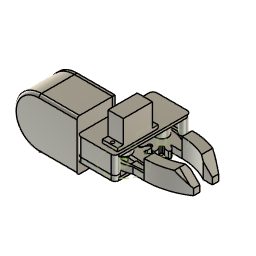
TRARM02_Link4_Gripper (Autodesk Fusion 360 design; units mm, degrees)
description: Spur Gear; Module: 2.5; Num Teeth: 12; Pressure Angle: 20.0; Backlash: 0.00 mm
Autodesk Fusion 360 part; units mm, degrees
(part 1 of 2)
sketch "스케치1" plane through (0, 0, 0) normal (0, 0, 1) x (1, 0, 0) in component "TRARM02_Link4A_30x40x2 v1"
  line L0 (20, 30) -> (20, 0)
  line L1 (-20, 30) -> (-20, 0)
  arc A0 (-20, 0) -> (20, 0) centre (0, 0) ccw
  line L2 (-20, 30) -> (20, 30)
  dimension "d1" = 40
  dimension "d128" = 30
  dimension "d129" = 20
  constraint coincident A0.centre origin
  constraint tangent L0 A0
  constraint vertical L0
  constraint parallel L0 L1
  constraint horizontal L0.start L1.start
  measures "d1" diameter of A0
  measures "d128" vertical distance of A0.centre L1.start
  measures "d129" distance of A0.centre L1
extrude "돌출1" add sketch "스케치1" along normal blind 2 makes body 1 in component "TRARM02_Link4A_30x40x2 v1"
sketch "스케치2" plane through (0, 0, 2) normal (0, 0, 1) x (-1, 0, 0) in component "TRARM02_Link4A_30x40x2 v1"
  circle A0 centre (0, 8.75) radius 1.1
  circle A1 centre (0, -19.05) radius 1.1
  line L0 (6.1, -16.65) -> (-6.1, -16.65)
  line L1 (-6.1, -16.65) -> (-6.1, 6.35)
  line L2 (-6.1, 6.35) -> (6.1, 6.35)
  line L3 (6.1, 6.35) -> (6.1, -16.65)
  dimension "d7" = 2.2
  dimension "d8" = 27.8
  dimension "d9" = 8.75
  dimension "d11" = 23
  dimension "d12" = 2.4
  dimension "d13" = 12.2
  dimension "d14" = 6.1
  constraint equal A0 A1
  constraint horizontal L0
  constraint vertical L1
  constraint horizontal L2
  constraint vertical L3
  constraint vertical origin A0.centre
  constraint vertical origin A1.centre
  measures "d7" diameter of A0
  measures "d8" distance of A0.centre A1.centre
  measures "d9" distance of origin A0.centre
  measures "d11" distance of L0.end L1.end
  measures "d12" vertical distance of A1.centre L0.end
  measures "d13" distance of L0.start L0.end
  measures "d14" horizontal distance of origin L1.end
extrude "돌출2" cut sketch "스케치2" against normal blind 2 bodies 1 in component "TRARM02_Link4A_30x40x2 v1"
chamfer "챔퍼2" distance 1.5 angle 45 2 edges at (1.0256, 19.4478, 0) (1.0256, -8.3522, 0) on bodies 1 in component "TRARM02_Link4A_30x40x2 v1"
sketch "스케치14" plane through (0, 0, 2) normal (0, 0, 1) x (-1, 0, 0) in component "TRARM02_Link4A_30x40x2 v1"
  line L0 (20, -30) -> (20, 0) construction
  line L1 (-20, 0) -> (-20, -30) construction
  arc A0 (20, 0) -> (-20, 0) centre (0, 0) ccw construction
  line L2 (19, -29) -> (19, 0)
  arc A1 (19, 0) -> (-19, 0) centre (0, 0) ccw
  line L3 (-19, 0) -> (-19, -29)
  line L4 (-15, -6) -> (-18, -6)
  line L5 (15, -6) -> (18, -6)
  line L6 (15, 0) -> (18, 0)
  arc A2 (15, 0) -> (15, -6) centre (15, -3) ccw
  line L7 (18, -28) -> (18, -6)
  line L8 (-18, -6) -> (-18, -28)
  line L9 (-15, 0) -> (-18, 0)
  arc A3 (18, 0) -> (-18, 0) centre (0, 0) ccw
  arc A4 (-15, -6) -> (-15, 0) centre (-15, -3) ccw
  line L10 (-20, -30) -> (20, -30)
  line L11 (18, -28) -> (-18, -28)
  line L12 (19, -29) -> (-19, -29)
  dimension "d112" = 3
  dimension "d113" = 3
  dimension "d120" = 3
  dimension "d121" = 1
  dimension "d124" = 6
  dimension "d125" = 6
  dimension "d126" = 3
  dimension "d130" = 1
  dimension "d131" = 1
  constraint coincident L6.end L7
  constraint perpendicular L6 L7
  constraint coincident L6 A2.start
  constraint horizontal L5
  constraint vertical L6.start A2.centre
  constraint coincident L6.start A2.start
  constraint horizontal L4
  constraint horizontal L9
  constraint vertical L8
  constraint equal L4 L9
  constraint vertical L4.end L9.end
  constraint coincident A0.centre L6
  constraint coincident A0.centre L9
  constraint concentric A0 A3
  constraint concentric A0 A1
  constraint tangent L2 A1
  constraint tangent A1 L3
  constraint vertical L7
  constraint horizontal L12
  constraint horizontal L11
  measures "d112" distance of L5.start L5.end
  measures "d113" distance of L4.start L4.end
  measures "d120" distance of L6.start L6.end
  measures "d121" distance of L3 L8
  measures "d124" distance of A0.centre L5
  measures "d125" distance of A0.centre L4
  measures "d126" radius of A4
  measures "d130" distance of L11 L12
  measures "d131" distance of L10 L12
extrude "돌출15" add sketch "스케치14" along normal blind 2 bodies 1 in component "TRARM02_Link4A_30x40x2 v1"
sketch "스케치16" plane through (0, 0, 4) normal (0, 0, 1) x (-1, 0, 0) in component "TRARM02_Link4A_30x40x2 v1"
  circle A0 centre (-15, -3) radius 1.5
  circle A1 centre (15, -3) radius 1.5
  arc A2 (15, 0) -> (15, -6) centre (15, -3) ccw
  arc A3 (-15, -6) -> (-15, 0) centre (-15, -3) ccw
  dimension "d106" = 3
  constraint equal A0 A1
  constraint concentric A1 A2
  constraint concentric A0 A3
  measures "d106" diameter of A0
extrude "돌출17" cut sketch "스케치16" against normal blind 4 bodies 1 in component "TRARM02_Link4A_30x40x2 v1"
chamfer "챔퍼4" distance 2 angle 45 1 edges at (16.3985, 3.5424, 0) on bodies 1 in component "TRARM02_Link4A_30x40x2 v1"
chamfer "챔퍼4" distance 2 angle 45 1 edges at (-13.6015, 3.5424, 0) on bodies 1 in component "TRARM02_Link4A_30x40x2 v1"
move_body "이동1" bodies 1 to x (0, -1, 0) y (1, 0, 0) z (0, 0, 1) at (0, 0, 0) in component "TRARM02_Link4A_30x40x2 v1"
sketch "스케치1 (2)" plane through (0, 0, 0) normal (0, 0, 1) x (1, 0, 0) in component "TRARM02_Link4B_30x40x28 v1"
  line L0 (20, 30) -> (20, 0)
  line L1 (-20, 30) -> (-20, 0)
  arc A0 (-20, 0) -> (20, 0) centre (0, 0) ccw
  line L2 (-20, 30) -> (20, 30)
  dimension "d1_1" = 40
  dimension "d144" = 30
  constraint coincident A0.centre origin
  constraint tangent L0 A0
  constraint vertical L0
  constraint parallel L0 L1
  constraint horizontal L0.start L1.start
  measures "d1_1" diameter of A0
  measures "d144" vertical distance of A0.centre L1.start
extrude "돌출1'" add sketch "스케치1 (2)" along normal blind 2 separate body makes body 2 in component "TRARM02_Link4B_30x40x28 v1"
sketch "스케치14 (2)" plane through (0, 0, 2) normal (0, 0, 1) x (-1, 0, 0) in component "TRARM02_Link4B_30x40x28 v1"
  line L0 (20, -30) -> (20, 0)
  line L1 (-20, 0) -> (-20, -30)
  arc A0 (20, 0) -> (-20, 0) centre (0, 0) ccw
  arc A1 (19, 0) -> (-19, 0) centre (0, 0) ccw
  line L2 (15, -6) -> (19, -6)
  line L3 (15, 0) -> (19, 0)
  arc A2 (15, 0) -> (15, -6) centre (15, -3) ccw
  line L4 (-15, -6) -> (-19, -6)
  arc A3 (-15, -6) -> (-15, 0) centre (-15, -3) ccw
  line L5 (19, -29) -> (19, -6)
  line L6 (-19, -6) -> (-19, -29)
  line L7 (-15, 0) -> (-19, 0)
  line L8 (-20, -30) -> (20, -30)
  line L9 (20, -30) -> (-20, -30)
  line L10 (19, -29) -> (-19, -29)
  dimension "d111_1" = 15
  dimension "d112_1" = 6
  dimension "d114" = 3
  dimension "d132" = 4
  dimension "d133" = 4
  dimension "d134" = 4
  dimension "d135" = 1
  dimension "d136" = 4
  dimension "d142" = 1
  dimension "d143" = 19
  dimension "d145" = 1
  constraint concentric A0 A1
  constraint equal A2 A3
  constraint horizontal A2.centre A3.centre
  constraint horizontal L7
  constraint vertical L6
  constraint horizontal L4
  constraint vertical L5
  constraint horizontal L3
  constraint coincident A1.start L3.end
  constraint horizontal L2
  constraint coincident L0.start L8.end
  constraint coincident L1.end L8.start
  constraint horizontal L10
  measures "d111_1" horizontal distance of A0.centre A2.centre
  measures "d112_1" diameter of A2
  measures "d114" vertical distance of A0.centre A2.centre
  measures "d132" distance of L3.start A1.start
  measures "d133" distance of L2.start L2.end
  measures "d134" distance of A1.end A3.end
  measures "d135" distance of L1 L6
  measures "d136" distance of L4.start L4.end
  measures "d142" distance of L0 L5
  measures "d143" radius of A1
  measures "d145" distance of L9 L10
extrude "돌출18" add sketch "스케치14 (2)" along normal blind 26 bodies 2 in component "TRARM02_Link4B_30x40x28 v1"
sketch "스케치17" plane through (0, 0, 28) normal (0, 0, 1) x (-1, 0, 0) in component "TRARM02_Link4B_30x40x28 v1"
  line L0 (-19, -6) -> (-15, -6)
  line L1 (-15, 0) -> (-19, 0)
  arc A0 (-15, -6) -> (-15, 0) centre (-15, -3) ccw
  arc A1 (15, 0) -> (15, -6) centre (15, -3) ccw
  line L2 (19, 0) -> (15, 0)
  line L3 (15, -6) -> (19, -6)
  line L4 (19, -6) -> (19, 0)
  line L5 (-19, -6) -> (-19, 0)
  point P0 (15, 0)
  constraint coincident L3.end L4.start
  constraint coincident L2.start L4.end
  constraint coincident L0.start L5.start
  constraint coincident L1.end L5.end
extrude "돌출19" cut sketch "스케치17" against normal blind 2 bodies 2 in component "TRARM02_Link4B_30x40x28 v1"
sketch "스케치18" plane through (0, 0, 26) normal (0, 0, 1) x (-1, 0, 0) in component "TRARM02_Link4B_30x40x28 v1"
  circle A0 centre (15, -3) radius 1.45
  arc A1 (15, 0) -> (15, -6) centre (15, -3) ccw
  circle A2 centre (-15, -3) radius 1.45
  arc A3 (-15, -6) -> (-15, 0) centre (-15, -3) ccw
  constraint concentric A0 A1
  constraint equal A0 A2
extrude "돌출20" cut sketch "스케치18" against normal blind 5 bodies 2 in component "TRARM02_Link4B_30x40x28 v1"
fillet "필렛4" radius 2 3 edges at (20, 15, 0) (0, -20, 0) (-20, 15, 0) on bodies 2 in component "TRARM02_Link4B_30x40x28 v1"
sketch "스케치20" plane through (0, 0, 0) normal (0, 1, 0) x (1, 0, 0) in component "TRARM02_Link4B_30x40x28 v1"
  circle A0 centre (0, -15) radius 5
  dimension "d146" = 10
  dimension "d147" = 15
  constraint vertical origin A0.centre
  measures "d146" diameter of A0
  measures "d147" distance of origin A0.centre
extrude "돌출22" cut sketch "스케치20" against normal blind 40 bodies 2 in component "TRARM02_Link4B_30x40x28 v1"
sketch "스케치21" plane through (0, 30, 0) normal (0, 1, 0) x (-1, 0, 0) in component "TRARM02_Link4B_30x40x28 v1"
  circle A0 centre (0, 10) radius 1.5
  circle A1 centre (0, 20) radius 1.5
  dimension "d153" = 3
  dimension "d159" = 10
  dimension "d160" = 10
  constraint vertical origin A0.centre
  constraint equal A0 A1
  constraint vertical origin A1.centre
  measures "d153" diameter of A0
  measures "d159" distance of origin A0.centre
  measures "d160" distance of A0.centre A1.centre
extrude "돌출23" cut sketch "스케치21" against normal blind 1 bodies 2 in component "TRARM02_Link4B_30x40x28 v1"
move_body "이동1'" bodies 2 to x (0, 0, -1) y (0, 1, 0) z (1, 0, 0) at (-30, 0, 30) in component "TRARM02_Link4B_30x40x28 v1"
move_body "이동2" bodies 1 to x (1, 0, 0) y (0, 0, 1) z (0, -1, 0) at (0, 0, 0) in component "TRARM02_Link4A_30x40x2 v1"
sketch "스케치1 (3)" plane through (0, 0, 0) normal (0, 0, 1) x (1, 0, 0) in component "TRGRIP01_Case_Bottom"
  line L0 (0, 0) -> (60, 0)
  line L1 (60, 0) -> (60, 30)
  line L2 (60, 30) -> (0, 30)
  line L3 (0, 30) -> (0, 0)
  dimension "d1_1_1" = 60
  dimension "d2_1" = 30
  constraint horizontal L0
  constraint vertical L1
  constraint horizontal L2
  constraint vertical L3
  constraint coincident L0.start L3.end
  measures "d1_1_1" distance of L0.start L0.end
  measures "d2_1" distance of L0.start L2.end
extrude "돌출1''" add sketch "스케치1 (3)" along normal blind 2 separate body makes body 3 in component "TRGRIP01_Case_Bottom"
sketch "스케치5" plane through (0, 0, 2) normal (0, 0, 1) x (-1, 0, 0) in component "TRGRIP01_Case_Bottom"
  line L0 (0, -30) -> (0, 0)
  line L1 (0, 0) -> (0, -30)
  line L2 (-60, -30) -> (0, -30)
  line L3 (-60, -30) -> (-60, 0)
  line L4 (0, 0) -> (-60, 0)
  line L5 (-60, 0) -> (-54, 0)
  line L6 (-54, -28) -> (-6, -28)
  line L7 (-2, -24) -> (-2, -6)
  line L8 (-6, 0) -> (0, 0)
  line L9 (-58, -24) -> (-58, -6)
  line L10 (-2, -24) -> (-6, -24)
  line L11 (-6, -24) -> (-6, -28)
  line L12 (-54, -28) -> (-54, -24)
  line L13 (-54, -24) -> (-58, -24)
  line L14 (-2, -6) -> (-6, -6)
  line L15 (0, 0) -> (-60, 0)
  line L16 (-6, -6) -> (-6, 0)
  line L17 (-58, -6) -> (-54, -6)
  line L18 (-54, -6) -> (-54, 0)
  point P0 (0, -30)
  point P1 (-60, -30)
  point P2 (-60, 0)
  dimension "d38" = 2
  dimension "d39" = 2
  dimension "d42" = 2
  dimension "d43" = 6
  dimension "d44" = 6
  dimension "d45" = 6
  dimension "d46" = 6
  dimension "d47" = 6
  constraint coincident L0.end L1.start
  constraint coincident P0 L0.start
  constraint coincident P1 L2.start
  constraint coincident P2 L3.end
  constraint coincident L4 L5.end
  constraint perpendicular L0 L5
  constraint perpendicular L0 L6
  constraint perpendicular L6 L7
  constraint perpendicular L1 L8
  constraint perpendicular L5 L9
  constraint perpendicular L7 L10
  constraint perpendicular L10 L11
  constraint perpendicular L6 L12
  constraint perpendicular L9 L13
  constraint perpendicular L7 L14
  constraint coincident L15 L8.start
  constraint perpendicular L15 L16
  constraint perpendicular L9 L17
  constraint perpendicular L4 L18
  constraint equal L10 L14
  constraint equal L11 L12
  constraint equal L13 L17
  measures "d38" distance of L2 L6
  measures "d39" distance of L3 L9
  measures "d42" distance of L1 L7
  measures "d43" distance of L0.end L8.start
  measures "d44" vertical distance of L0.end L14.end
  measures "d45" distance of P2 L5.end
  measures "d46" distance of L17.end L5.end
  measures "d47" vertical distance of P0 L10.end
extrude "돌출11" add sketch "스케치5" along normal blind 2 contours L0 L1 L2 L3 L4 L5 L6 L7 L8 L9 L10 L11 L12 L13 L14 L15 L16 L17 L18 bodies 3 in component "TRGRIP01_Case_Bottom"
sketch "스케치10" plane through (0, 0, 4) normal (0, 0, 1) x (-1, 0, 0) in component "TRGRIP01_Case_Bottom"
  circle A0 centre (-57, -3) radius 1
  circle A1 centre (-57, -27) radius 1
  circle A2 centre (-3, -3) radius 1
  circle A3 centre (-3, -27) radius 1
  dimension "d82" = 2
  dimension "d83" = 3
  dimension "d84" = 3
  dimension "d85" = 24
  dimension "d86" = 54
  constraint equal A2 A3
  constraint equal A1 A2
  constraint equal A0 A1
  constraint vertical A2.centre A3.centre
  constraint horizontal A0.centre A2.centre
  constraint vertical A0.centre A1.centre
  constraint horizontal A1.centre A3.centre
  measures "d82" diameter of A0
  measures "d83" horizontal distance of origin A2.centre
  measures "d84" vertical distance of origin A2.centre
  measures "d85" distance of A2.centre A3.centre
  measures "d86" distance of A0.centre A2.centre
extrude "돌출13" cut sketch "스케치10" against normal blind 4 bodies 3 in component "TRGRIP01_Case_Bottom"
fillet "필렛4'" radius 3 10 edges at (0, 0, 2) (60, 0, 2) (0, 30, 2) (60, 30, 2) (54, 24, 3) (6, 24, 3) (6, 6, 3) (54, 6, 3) (6, 0, 3) (54, 0, 3) on bodies 3 in component "TRGRIP01_Case_Bottom"
chamfer "챔퍼1" distance 1.5 angle 45 4 edges at (57.9323, 3.3616, 0) (57.9323, 27.3616, 0) (3.9323, 27.3616, 0) (3.9323, 3.3616, 0) on bodies 3 in component "TRGRIP01_Case_Bottom"
sketch "스케치11" plane through (0, 0, 2) normal (0, 0, 1) x (-1, 0, 0) in component "TRGRIP01_Case_Bottom"
  circle A0 centre (-45, -8.1) radius 2.3
  circle A1 centre (-15, -8.1) radius 2.3
  dimension "d93" = 8.1
  dimension "d95" = 4.6
  dimension "d98" = 15
  dimension "d99" = 30
  constraint equal A0 A1
  constraint horizontal A0.centre A1.centre
  measures "d93" vertical distance of origin A0.centre
  measures "d95" diameter of A0
  measures "d98" horizontal distance of origin A1.centre
  measures "d99" distance of A0.centre A1.centre
extrude "돌출14" add sketch "스케치11" along normal blind 1.5 bodies 3 in component "TRGRIP01_Case_Bottom"
sketch "스케치1 (4)" plane through (0, 0, 0) normal (0, 0, 1) x (1, 0, 0) in component "Spur Gear (12 teeth)"
  circle A0 centre (0, 0) radius 11.9492
  circle A1 centre (0, 0) radius 2.5
sketch "스케치2 (2)" plane through (0, 0, 0) normal (0, 0, 1) x (1, 0, 0) in component "Spur Gear (12 teeth)"
  spline S0 degree 5 poles (13.9458, -2.0479) (13.9559, -2.0494) (13.9759, -2.052) (14.0061, -2.0549) (14.0465, -2.057) (14.0972, -2.0572) (14.1481, -2.0556) (14.199, -2.0528) (14.2501, -2.0495) (14.3011, -2.0457) (14.3522, -2.0415) (14.4034, -2.0367) (14.4546, -2.0311) (14.5058, -2.0247) (14.5571, -2.0173) (14.6084, -2.0091) (14.6597, -2.0003) (14.7111, -1.9908) (14.7624, -1.9808) (14.8137, -1.9703) (14.8651, -1.9594) (14.9164, -1.9479) (14.9678, -1.9358) (15.0191, -1.9232) (15.0705, -1.91) (15.1218, -1.8963) (15.1731, -1.882) (15.2244, -1.8673) (15.2757, -1.8521) (15.3269, -1.8365) (15.3781, -1.8204) (15.4293, -1.8038) (15.4805, -1.7868) (15.5316, -1.7693) (15.5827, -1.7513) (15.6338, -1.7329) (15.6848, -1.7141) (15.7358, -1.6948) (15.7868, -1.6751) (15.8377, -1.655) (15.8886, -1.6345) (15.9394, -1.6136) (15.9902, -1.5922) (16.0409, -1.5705) (16.0916, -1.5483) (16.1422, -1.5258) (16.1928, -1.5028) (16.2433, -1.4794) (16.2937, -1.4557) (16.3441, -1.4316) (16.3944, -1.4071) (16.4447, -1.3822) (16.4949, -1.3569) (16.545, -1.3313) (16.5951, -1.3053) (16.6451, -1.2789) (16.695, -1.2521) (16.7448, -1.225) (16.7946, -1.1975) (16.8443, -1.1697) (16.8939, -1.1415) (16.9435, -1.1129) (16.9929, -1.084) (17.0423, -1.0548) (17.0916, -1.0251) (17.1408, -0.9952) (17.1899, -0.9649) (17.239, -0.9343) (17.2879, -0.9033) (17.3368, -0.8719) (17.3856, -0.8403) (17.4245, -0.8147) (17.4537, -0.7953) (17.4731, -0.7824) (17.4828, -0.7759) knots 0 0 0 0 0 0 0.01428571 0.02857143 0.04285714 0.05714286 0.07142857 0.08571429 0.1 0.11428571 0.12857143 0.14285714 0.15714286 0.17142857 0.18571429 0.2 0.21428571 0.22857143 0.24285714 0.25714286 0.27142857 0.28571429 0.3 0.31428571 0.32857143 0.34285714 0.35714286 0.37142857 0.38571429 0.4 0.41428571 0.42857143 0.44285714 0.45714286 0.47142857 0.48571429 0.5 0.51428571 0.52857143 0.54285714 0.55714286 0.57142857 0.58571429 0.6 0.61428571 0.62857143 0.64285714 0.65714286 0.67142857 0.68571429 0.7 0.71428571 0.72857143 0.74285714 0.75714286 0.77142857 0.78571429 0.8 0.81428571 0.82857143 0.84285714 0.85714286 0.87142857 0.88571429 0.9 0.91428571 0.92857143 0.94285714 0.95714286 0.97142857 0.98571429 1 1 1 1 1 1
  spline S1 degree 5 poles (13.9458, 2.0479) (13.9559, 2.0494) (13.9759, 2.052) (14.0061, 2.0549) (14.0465, 2.057) (14.0972, 2.0572) (14.1481, 2.0556) (14.199, 2.0528) (14.2501, 2.0495) (14.3011, 2.0457) (14.3522, 2.0415) (14.4034, 2.0367) (14.4546, 2.0311) (14.5058, 2.0247) (14.5571, 2.0173) (14.6084, 2.0091) (14.6597, 2.0003) (14.7111, 1.9908) (14.7624, 1.9808) (14.8137, 1.9703) (14.8651, 1.9594) (14.9164, 1.9479) (14.9678, 1.9358) (15.0191, 1.9232) (15.0705, 1.91) (15.1218, 1.8963) (15.1731, 1.882) (15.2244, 1.8673) (15.2757, 1.8521) (15.3269, 1.8365) (15.3781, 1.8204) (15.4293, 1.8038) (15.4805, 1.7868) (15.5316, 1.7693) (15.5827, 1.7513) (15.6338, 1.7329) (15.6848, 1.7141) (15.7358, 1.6948) (15.7868, 1.6751) (15.8377, 1.655) (15.8886, 1.6345) (15.9394, 1.6136) (15.9902, 1.5922) (16.0409, 1.5705) (16.0916, 1.5483) (16.1422, 1.5258) (16.1928, 1.5028) (16.2433, 1.4794) (16.2937, 1.4557) (16.3441, 1.4316) (16.3944, 1.4071) (16.4447, 1.3822) (16.4949, 1.3569) (16.545, 1.3313) (16.5951, 1.3053) (16.6451, 1.2789) (16.695, 1.2521) (16.7448, 1.225) (16.7946, 1.1975) (16.8443, 1.1697) (16.8939, 1.1415) (16.9435, 1.1129) (16.9929, 1.084) (17.0423, 1.0548) (17.0916, 1.0251) (17.1408, 0.9952) (17.1899, 0.9649) (17.239, 0.9343) (17.2879, 0.9033) (17.3368, 0.8719) (17.3856, 0.8403) (17.4245, 0.8147) (17.4537, 0.7953) (17.4731, 0.7824) (17.4828, 0.7759) knots 0 0 0 0 0 0 0.01428571 0.02857143 0.04285714 0.05714286 0.07142857 0.08571429 0.1 0.11428571 0.12857143 0.14285714 0.15714286 0.17142857 0.18571429 0.2 0.21428571 0.22857143 0.24285714 0.25714286 0.27142857 0.28571429 0.3 0.31428571 0.32857143 0.34285714 0.35714286 0.37142857 0.38571429 0.4 0.41428571 0.42857143 0.44285714 0.45714286 0.47142857 0.48571429 0.5 0.51428571 0.52857143 0.54285714 0.55714286 0.57142857 0.58571429 0.6 0.61428571 0.62857143 0.64285714 0.65714286 0.67142857 0.68571429 0.7 0.71428571 0.72857143 0.74285714 0.75714286 0.77142857 0.78571429 0.8 0.81428571 0.82857143 0.84285714 0.85714286 0.87142857 0.88571429 0.9 0.91428571 0.92857143 0.94285714 0.95714286 0.97142857 0.98571429 1 1 1 1 1 1
  arc A0 (17.4828, -0.7759) -> (17.4828, 0.7759) centre (0, 0) ccw
  line L0 (11.8125, -1.7361) -> (13.9458, -2.0479)
  line L1 (11.8125, 1.7361) -> (13.9458, 2.0479)
  line L2 (11.8125, -1.7361) -> (11.8125, 1.7361)
  point P0 (14.1908, -2.0531)
  point P1 (14.4394, -2.0327)
  point P2 (14.6902, -1.9946)
  point P3 (14.9425, -1.9417)
  point P4 (15.196, -1.8754)
  point P5 (15.4504, -1.7967)
  point P6 (15.7053, -1.7063)
  point P7 (15.9604, -1.6047)
  point P8 (16.2156, -1.4922)
  point P9 (16.4704, -1.3692)
  point P10 (16.7248, -1.2358)
  point P11 (16.9785, -1.0924)
  point P12 (17.2312, -0.939)
  point P13 (14.1908, 2.0531)
  point P14 (14.4394, 2.0327)
  point P15 (14.6902, 1.9946)
  point P16 (14.9425, 1.9417)
  point P17 (15.196, 1.8754)
  point P18 (15.4504, 1.7967)
  point P19 (15.7053, 1.7063)
  point P20 (15.9604, 1.6047)
  point P21 (16.2156, 1.4922)
  point P22 (16.4704, 1.3692)
  point P23 (16.7248, 1.2358)
  point P24 (16.9785, 1.0924)
  point P25 (17.2312, 0.939)
sketch "스케치3" plane through (0, 0, 0) normal (0, 0, 1) x (1, 0, 0) in component "Spur Gear (12 teeth)"
sketch "스케치1 (5)" plane through (0, 0, 0) normal (0, 0, 1) x (1, 0, 0) in component "Spur Gear (12 teeth) (1)"
  circle A0 centre (0, 0) radius 11.9492
  circle A1 centre (0, 0) radius 2.5
  dimension "d44_1" = 5
  measures "d44_1" diameter of A1
extrude "돌출1'''" add sketch "스케치1 (5)" along normal blind 5 separate body makes body 4 in component "Spur Gear (12 teeth) (1)"
sketch "스케치2 (3)" plane through (0, 0, 0) normal (0, 0, 1) x (1, 0, 0) in component "Spur Gear (12 teeth) (1)"
  spline S0 degree 5 poles (13.9458, -2.0479) (13.9559, -2.0494) (13.9759, -2.052) (14.0061, -2.0549) (14.0465, -2.057) (14.0972, -2.0572) (14.1481, -2.0556) (14.199, -2.0528) (14.2501, -2.0495) (14.3011, -2.0457) (14.3522, -2.0415) (14.4034, -2.0367) (14.4546, -2.0311) (14.5058, -2.0247) (14.5571, -2.0173) (14.6084, -2.0091) (14.6597, -2.0003) (14.7111, -1.9908) (14.7624, -1.9808) (14.8137, -1.9703) (14.8651, -1.9594) (14.9164, -1.9479) (14.9678, -1.9358) (15.0191, -1.9232) (15.0705, -1.91) (15.1218, -1.8963) (15.1731, -1.882) (15.2244, -1.8673) (15.2757, -1.8521) (15.3269, -1.8365) (15.3781, -1.8204) (15.4293, -1.8038) (15.4805, -1.7868) (15.5316, -1.7693) (15.5827, -1.7513) (15.6338, -1.7329) (15.6848, -1.7141) (15.7358, -1.6948) (15.7868, -1.6751) (15.8377, -1.655) (15.8886, -1.6345) (15.9394, -1.6136) (15.9902, -1.5922) (16.0409, -1.5705) (16.0916, -1.5483) (16.1422, -1.5258) (16.1928, -1.5028) (16.2433, -1.4794) (16.2937, -1.4557) (16.3441, -1.4316) (16.3944, -1.4071) (16.4447, -1.3822) (16.4949, -1.3569) (16.545, -1.3313) (16.5951, -1.3053) (16.6451, -1.2789) (16.695, -1.2521) (16.7448, -1.225) (16.7946, -1.1975) (16.8443, -1.1697) (16.8939, -1.1415) (16.9435, -1.1129) (16.9929, -1.084) (17.0423, -1.0548) (17.0916, -1.0251) (17.1408, -0.9952) (17.1899, -0.9649) (17.239, -0.9343) (17.2879, -0.9033) (17.3368, -0.8719) (17.3856, -0.8403) (17.4245, -0.8147) (17.4537, -0.7953) (17.4731, -0.7824) (17.4828, -0.7759) knots 0 0 0 0 0 0 0.01428571 0.02857143 0.04285714 0.05714286 0.07142857 0.08571429 0.1 0.11428571 0.12857143 0.14285714 0.15714286 0.17142857 0.18571429 0.2 0.21428571 0.22857143 0.24285714 0.25714286 0.27142857 0.28571429 0.3 0.31428571 0.32857143 0.34285714 0.35714286 0.37142857 0.38571429 0.4 0.41428571 0.42857143 0.44285714 0.45714286 0.47142857 0.48571429 0.5 0.51428571 0.52857143 0.54285714 0.55714286 0.57142857 0.58571429 0.6 0.61428571 0.62857143 0.64285714 0.65714286 0.67142857 0.68571429 0.7 0.71428571 0.72857143 0.74285714 0.75714286 0.77142857 0.78571429 0.8 0.81428571 0.82857143 0.84285714 0.85714286 0.87142857 0.88571429 0.9 0.91428571 0.92857143 0.94285714 0.95714286 0.97142857 0.98571429 1 1 1 1 1 1
  spline S1 degree 5 poles (13.9458, 2.0479) (13.9559, 2.0494) (13.9759, 2.052) (14.0061, 2.0549) (14.0465, 2.057) (14.0972, 2.0572) (14.1481, 2.0556) (14.199, 2.0528) (14.2501, 2.0495) (14.3011, 2.0457) (14.3522, 2.0415) (14.4034, 2.0367) (14.4546, 2.0311) (14.5058, 2.0247) (14.5571, 2.0173) (14.6084, 2.0091) (14.6597, 2.0003) (14.7111, 1.9908) (14.7624, 1.9808) (14.8137, 1.9703) (14.8651, 1.9594) (14.9164, 1.9479) (14.9678, 1.9358) (15.0191, 1.9232) (15.0705, 1.91) (15.1218, 1.8963) (15.1731, 1.882) (15.2244, 1.8673) (15.2757, 1.8521) (15.3269, 1.8365) (15.3781, 1.8204) (15.4293, 1.8038) (15.4805, 1.7868) (15.5316, 1.7693) (15.5827, 1.7513) (15.6338, 1.7329) (15.6848, 1.7141) (15.7358, 1.6948) (15.7868, 1.6751) (15.8377, 1.655) (15.8886, 1.6345) (15.9394, 1.6136) (15.9902, 1.5922) (16.0409, 1.5705) (16.0916, 1.5483) (16.1422, 1.5258) (16.1928, 1.5028) (16.2433, 1.4794) (16.2937, 1.4557) (16.3441, 1.4316) (16.3944, 1.4071) (16.4447, 1.3822) (16.4949, 1.3569) (16.545, 1.3313) (16.5951, 1.3053) (16.6451, 1.2789) (16.695, 1.2521) (16.7448, 1.225) (16.7946, 1.1975) (16.8443, 1.1697) (16.8939, 1.1415) (16.9435, 1.1129) (16.9929, 1.084) (17.0423, 1.0548) (17.0916, 1.0251) (17.1408, 0.9952) (17.1899, 0.9649) (17.239, 0.9343) (17.2879, 0.9033) (17.3368, 0.8719) (17.3856, 0.8403) (17.4245, 0.8147) (17.4537, 0.7953) (17.4731, 0.7824) (17.4828, 0.7759) knots 0 0 0 0 0 0 0.01428571 0.02857143 0.04285714 0.05714286 0.07142857 0.08571429 0.1 0.11428571 0.12857143 0.14285714 0.15714286 0.17142857 0.18571429 0.2 0.21428571 0.22857143 0.24285714 0.25714286 0.27142857 0.28571429 0.3 0.31428571 0.32857143 0.34285714 0.35714286 0.37142857 0.38571429 0.4 0.41428571 0.42857143 0.44285714 0.45714286 0.47142857 0.48571429 0.5 0.51428571 0.52857143 0.54285714 0.55714286 0.57142857 0.58571429 0.6 0.61428571 0.62857143 0.64285714 0.65714286 0.67142857 0.68571429 0.7 0.71428571 0.72857143 0.74285714 0.75714286 0.77142857 0.78571429 0.8 0.81428571 0.82857143 0.84285714 0.85714286 0.87142857 0.88571429 0.9 0.91428571 0.92857143 0.94285714 0.95714286 0.97142857 0.98571429 1 1 1 1 1 1
  arc A0 (17.4828, -0.7759) -> (17.4828, 0.7759) centre (0, 0) ccw
  line L0 (11.8125, -1.7361) -> (13.9458, -2.0479)
  line L1 (11.8125, 1.7361) -> (13.9458, 2.0479)
  line L2 (11.8125, -1.7361) -> (11.8125, 1.7361)
  point P0 (14.1908, -2.0531)
  point P1 (14.4394, -2.0327)
  point P2 (14.6902, -1.9946)
  point P3 (14.9425, -1.9417)
  point P4 (15.196, -1.8754)
  point P5 (15.4504, -1.7967)
  point P6 (15.7053, -1.7063)
  point P7 (15.9604, -1.6047)
  point P8 (16.2156, -1.4922)
  point P9 (16.4704, -1.3692)
  point P10 (16.7248, -1.2358)
  point P11 (16.9785, -1.0924)
  point P12 (17.2312, -0.939)
  point P13 (14.1908, 2.0531)
  point P14 (14.4394, 2.0327)
  point P15 (14.6902, 1.9946)
  point P16 (14.9425, 1.9417)
  point P17 (15.196, 1.8754)
  point P18 (15.4504, 1.7967)
  point P19 (15.7053, 1.7063)
  point P20 (15.9604, 1.6047)
  point P21 (16.2156, 1.4922)
  point P22 (16.4704, 1.3692)
  point P23 (16.7248, 1.2358)
  point P24 (16.9785, 1.0924)
  point P25 (17.2312, 0.939)
extrude "돌출2'" add sketch "스케치2 (3)" along normal blind 5 bodies 4 in component "Spur Gear (12 teeth) (1)"
fillet "필렛1" radius 1 2 edges at (11.8222, -1.7375, 2.5) (11.8222, 1.7375, 2.5) on bodies 4 in component "Spur Gear (12 teeth) (1)"
pattern_circular "C-패턴1" count 7 over 180 about axis through (0, 0, 0) along (0, 0, 1) of "돌출2'", "필렛1" in component "Spur Gear (12 teeth) (1)"
sketch "스케치3 (2)" plane through (0, 0, 0) normal (0, 0, 1) x (1, 0, 0) in component "Spur Gear (12 teeth) (1)"
  circle A0 centre (0, 0) radius 15 construction
sketch "스케치1 (6)" plane through (0, 0, 0) normal (0, 0, 1) x (1, 0, 0) in component "TRGRIP01_GearLink_Left"
  line L0 (-50, 4) -> (-10, 4)
  line L1 (-10, 4) -> (-10, -4)
  line L2 (-10, -4) -> (-50, -4)
  line L3 (-50, -4) -> (-50, 4)
  dimension "d25" = 8
  dimension "d26" = 40
  dimension "d27" = 4
  dimension "d28" = 50
  constraint horizontal L0
  constraint vertical L1
  constraint horizontal L2
  constraint vertical L3
  measures "d25" distance of L0.start L2.end
  measures "d26" distance of L1.end L2.end
  measures "d27" vertical distance of origin L0.start
  measures "d28" distance of origin L3
extrude "돌출3" add sketch "스케치1 (6)" along normal blind 15 bodies 4 in component "Spur Gear (12 teeth) (1)"
extrude "돌출7" cut 1 faces at (-10, 1.3333, 8.3333) along direction (-1, 0, 0) blind 10 on bodies 4 bodies 4 in component "Spur Gear (12 teeth) (1)"
sketch "스케치4" plane through (0, 4, 0) normal (0, 1, 0) x (-1, 0, 0) in component "TRGRIP01_GearLink_Left"
  line L0 (20, 15) -> (50, 15)
  line L1 (50, 15) -> (50, 0)
  line L2 (50, 0) -> (20, 0)
  line L3 (20, 0) -> (20, 15)
  point P0 (20, 15)
  point P1 (50, 0)
  constraint horizontal L0
  constraint vertical L1
  constraint horizontal L2
  constraint vertical L3
  constraint coincident P1 L1.end
  constraint coincident P0 L0.start
extrude "돌출8" add sketch "스케치4" along normal blind 6 bodies 4 in component "Spur Gear (12 teeth) (1)"
chamfer "챔퍼1'" distance 10 angle 45 1 edges at (-50, 0, 15) on bodies 4 in component "Spur Gear (12 teeth) (1)"
sketch "스케치3 (3)" plane through (0, 0, 5) normal (0, 0, 1) x (-1, 0, 0) in component "TRGRIP01_GearLink_Left"
  arc A0 (11.2598, 4) -> (-11.6529, 2.6446) centre (0, 0) ccw
  arc A1 (11.2598, 4) -> (-11.6529, 2.6446) centre (0, 0) ccw
  circle A2 centre (0, -20) radius 26.5101
  dimension "d50" = 20
  constraint vertical A0.centre A2.centre
  constraint coincident A0.start A2
  measures "d50" distance of A0.centre A2.centre
extrude "돌출10" cut sketch "스케치3 (3)" against normal blind 5 contours A0 A1 A2 bodies 4 in component "Spur Gear (12 teeth) (1)"
sketch "스케치5 (2)" plane through (0, 0, 0) normal (0, 0, -1) x (1, 0, 0) in component "TRGRIP01_GearLink_Left"
  line L0 (-20, -10) -> (-50, -10)
  line L1 (-50, -10) -> (-20, -10)
  circle A0 centre (-20, -50) radius 46
  circle A1 centre (-20, -50) radius 54
  line L2 (-20, -10) -> (-20, -4)
  line L3 (-20, -10) -> (-42.7156, -10)
  line L4 (-20, 4) -> (-50, 4)
  line L5 (-50, 4) -> (-50, -5.1001)
  point P0 (-50, -10)
  point P1 (-20, -10)
  point P2 (-20, -4)
  point P3 (-20, 4)
  dimension "d61" = 20
  dimension "d62" = 50
  constraint coincident A0 P2
  constraint concentric A0 A1
  constraint coincident A1 P3
  constraint coincident P1 L0.start
  constraint coincident P2 L2.end
  constraint coincident L0 L3.end
  constraint coincident A0 L3.end
  constraint perpendicular L2 L3
  constraint coincident P3 L4.start
  constraint tangent A1 L4
  constraint horizontal L4
  constraint coincident A1 L5.end
  constraint perpendicular L4 L5
  measures "d61" horizontal distance of origin A0.centre
  measures "d62" vertical distance of origin A0.centre
extrude "돌출13'" cut sketch "스케치5 (2)" against normal blind 15 contours L0 L1 A0 L2 L3 | A1 L4 L5 picked at (-21.9743, -6.1276) bodies 4 in component "Spur Gear (12 teeth) (1)"
sketch "스케치1 (7)" plane through (0, 0, 0) normal (0, 0, 1) x (1, 0, 0) in component "Spur Gear (12 teeth) (2)"
  circle A0 centre (0, 0) radius 11.9492
  circle A1 centre (0, 0) radius 2.5
sketch "스케치2 (4)" plane through (0, 0, 0) normal (0, 0, 1) x (1, 0, 0) in component "Spur Gear (12 teeth) (2)"
  spline S0 degree 5 poles (13.9458, -2.0479) (13.9559, -2.0494) (13.9759, -2.052) (14.0061, -2.0549) (14.0465, -2.057) (14.0972, -2.0572) (14.1481, -2.0556) (14.199, -2.0528) (14.2501, -2.0495) (14.3011, -2.0457) (14.3522, -2.0415) (14.4034, -2.0367) (14.4546, -2.0311) (14.5058, -2.0247) (14.5571, -2.0173) (14.6084, -2.0091) (14.6597, -2.0003) (14.7111, -1.9908) (14.7624, -1.9808) (14.8137, -1.9703) (14.8651, -1.9594) (14.9164, -1.9479) (14.9678, -1.9358) (15.0191, -1.9232) (15.0705, -1.91) (15.1218, -1.8963) (15.1731, -1.882) (15.2244, -1.8673) (15.2757, -1.8521) (15.3269, -1.8365) (15.3781, -1.8204) (15.4293, -1.8038) (15.4805, -1.7868) (15.5316, -1.7693) (15.5827, -1.7513) (15.6338, -1.7329) (15.6848, -1.7141) (15.7358, -1.6948) (15.7868, -1.6751) (15.8377, -1.655) (15.8886, -1.6345) (15.9394, -1.6136) (15.9902, -1.5922) (16.0409, -1.5705) (16.0916, -1.5483) (16.1422, -1.5258) (16.1928, -1.5028) (16.2433, -1.4794) (16.2937, -1.4557) (16.3441, -1.4316) (16.3944, -1.4071) (16.4447, -1.3822) (16.4949, -1.3569) (16.545, -1.3313) (16.5951, -1.3053) (16.6451, -1.2789) (16.695, -1.2521) (16.7448, -1.225) (16.7946, -1.1975) (16.8443, -1.1697) (16.8939, -1.1415) (16.9435, -1.1129) (16.9929, -1.084) (17.0423, -1.0548) (17.0916, -1.0251) (17.1408, -0.9952) (17.1899, -0.9649) (17.239, -0.9343) (17.2879, -0.9033) (17.3368, -0.8719) (17.3856, -0.8403) (17.4245, -0.8147) (17.4537, -0.7953) (17.4731, -0.7824) (17.4828, -0.7759) knots 0 0 0 0 0 0 0.01428571 0.02857143 0.04285714 0.05714286 0.07142857 0.08571429 0.1 0.11428571 0.12857143 0.14285714 0.15714286 0.17142857 0.18571429 0.2 0.21428571 0.22857143 0.24285714 0.25714286 0.27142857 0.28571429 0.3 0.31428571 0.32857143 0.34285714 0.35714286 0.37142857 0.38571429 0.4 0.41428571 0.42857143 0.44285714 0.45714286 0.47142857 0.48571429 0.5 0.51428571 0.52857143 0.54285714 0.55714286 0.57142857 0.58571429 0.6 0.61428571 0.62857143 0.64285714 0.65714286 0.67142857 0.68571429 0.7 0.71428571 0.72857143 0.74285714 0.75714286 0.77142857 0.78571429 0.8 0.81428571 0.82857143 0.84285714 0.85714286 0.87142857 0.88571429 0.9 0.91428571 0.92857143 0.94285714 0.95714286 0.97142857 0.98571429 1 1 1 1 1 1
  spline S1 degree 5 poles (13.9458, 2.0479) (13.9559, 2.0494) (13.9759, 2.052) (14.0061, 2.0549) (14.0465, 2.057) (14.0972, 2.0572) (14.1481, 2.0556) (14.199, 2.0528) (14.2501, 2.0495) (14.3011, 2.0457) (14.3522, 2.0415) (14.4034, 2.0367) (14.4546, 2.0311) (14.5058, 2.0247) (14.5571, 2.0173) (14.6084, 2.0091) (14.6597, 2.0003) (14.7111, 1.9908) (14.7624, 1.9808) (14.8137, 1.9703) (14.8651, 1.9594) (14.9164, 1.9479) (14.9678, 1.9358) (15.0191, 1.9232) (15.0705, 1.91) (15.1218, 1.8963) (15.1731, 1.882) (15.2244, 1.8673) (15.2757, 1.8521) (15.3269, 1.8365) (15.3781, 1.8204) (15.4293, 1.8038) (15.4805, 1.7868) (15.5316, 1.7693) (15.5827, 1.7513) (15.6338, 1.7329) (15.6848, 1.7141) (15.7358, 1.6948) (15.7868, 1.6751) (15.8377, 1.655) (15.8886, 1.6345) (15.9394, 1.6136) (15.9902, 1.5922) (16.0409, 1.5705) (16.0916, 1.5483) (16.1422, 1.5258) (16.1928, 1.5028) (16.2433, 1.4794) (16.2937, 1.4557) (16.3441, 1.4316) (16.3944, 1.4071) (16.4447, 1.3822) (16.4949, 1.3569) (16.545, 1.3313) (16.5951, 1.3053) (16.6451, 1.2789) (16.695, 1.2521) (16.7448, 1.225) (16.7946, 1.1975) (16.8443, 1.1697) (16.8939, 1.1415) (16.9435, 1.1129) (16.9929, 1.084) (17.0423, 1.0548) (17.0916, 1.0251) (17.1408, 0.9952) (17.1899, 0.9649) (17.239, 0.9343) (17.2879, 0.9033) (17.3368, 0.8719) (17.3856, 0.8403) (17.4245, 0.8147) (17.4537, 0.7953) (17.4731, 0.7824) (17.4828, 0.7759) knots 0 0 0 0 0 0 0.01428571 0.02857143 0.04285714 0.05714286 0.07142857 0.08571429 0.1 0.11428571 0.12857143 0.14285714 0.15714286 0.17142857 0.18571429 0.2 0.21428571 0.22857143 0.24285714 0.25714286 0.27142857 0.28571429 0.3 0.31428571 0.32857143 0.34285714 0.35714286 0.37142857 0.38571429 0.4 0.41428571 0.42857143 0.44285714 0.45714286 0.47142857 0.48571429 0.5 0.51428571 0.52857143 0.54285714 0.55714286 0.57142857 0.58571429 0.6 0.61428571 0.62857143 0.64285714 0.65714286 0.67142857 0.68571429 0.7 0.71428571 0.72857143 0.74285714 0.75714286 0.77142857 0.78571429 0.8 0.81428571 0.82857143 0.84285714 0.85714286 0.87142857 0.88571429 0.9 0.91428571 0.92857143 0.94285714 0.95714286 0.97142857 0.98571429 1 1 1 1 1 1
  arc A0 (17.4828, -0.7759) -> (17.4828, 0.7759) centre (0, 0) ccw
  line L0 (11.8125, -1.7361) -> (13.9458, -2.0479)
  line L1 (11.8125, 1.7361) -> (13.9458, 2.0479)
  line L2 (11.8125, -1.7361) -> (11.8125, 1.7361)
  point P0 (14.1908, -2.0531)
  point P1 (14.4394, -2.0327)
  point P2 (14.6902, -1.9946)
  point P3 (14.9425, -1.9417)
  point P4 (15.196, -1.8754)
  point P5 (15.4504, -1.7967)
  point P6 (15.7053, -1.7063)
  point P7 (15.9604, -1.6047)
  point P8 (16.2156, -1.4922)
  point P9 (16.4704, -1.3692)
  point P10 (16.7248, -1.2358)
  point P11 (16.9785, -1.0924)
  point P12 (17.2312, -0.939)
  point P13 (14.1908, 2.0531)
  point P14 (14.4394, 2.0327)
  point P15 (14.6902, 1.9946)
  point P16 (14.9425, 1.9417)
  point P17 (15.196, 1.8754)
  point P18 (15.4504, 1.7967)
  point P19 (15.7053, 1.7063)
  point P20 (15.9604, 1.6047)
  point P21 (16.2156, 1.4922)
  point P22 (16.4704, 1.3692)
  point P23 (16.7248, 1.2358)
  point P24 (16.9785, 1.0924)
  point P25 (17.2312, 0.939)
sketch "스케치3 (4)" plane through (0, 0, 0) normal (0, 0, 1) x (1, 0, 0) in component "Spur Gear (12 teeth) (2)"
sketch "스케치1 (8)" plane through (0, 0, 0) normal (0, 0, 1) x (1, 0, 0) in component "Spur Gear (12 teeth) (1) (1)"
  circle A0 centre (0, 0) radius 11.9492
  circle A1 centre (0, 0) radius 2.5
extrude "돌출1''''" add sketch "스케치1 (8)" along normal blind 5 separate body makes body 5 in component "Spur Gear (12 teeth) (1) (1)"
sketch "스케치2 (5)" plane through (0, 0, 0) normal (0, 0, 1) x (1, 0, 0) in component "Spur Gear (12 teeth) (1) (1)"
  spline S0 degree 5 poles (13.9458, -2.0479) (13.9559, -2.0494) (13.9759, -2.052) (14.0061, -2.0549) (14.0465, -2.057) (14.0972, -2.0572) (14.1481, -2.0556) (14.199, -2.0528) (14.2501, -2.0495) (14.3011, -2.0457) (14.3522, -2.0415) (14.4034, -2.0367) (14.4546, -2.0311) (14.5058, -2.0247) (14.5571, -2.0173) (14.6084, -2.0091) (14.6597, -2.0003) (14.7111, -1.9908) (14.7624, -1.9808) (14.8137, -1.9703) (14.8651, -1.9594) (14.9164, -1.9479) (14.9678, -1.9358) (15.0191, -1.9232) (15.0705, -1.91) (15.1218, -1.8963) (15.1731, -1.882) (15.2244, -1.8673) (15.2757, -1.8521) (15.3269, -1.8365) (15.3781, -1.8204) (15.4293, -1.8038) (15.4805, -1.7868) (15.5316, -1.7693) (15.5827, -1.7513) (15.6338, -1.7329) (15.6848, -1.7141) (15.7358, -1.6948) (15.7868, -1.6751) (15.8377, -1.655) (15.8886, -1.6345) (15.9394, -1.6136) (15.9902, -1.5922) (16.0409, -1.5705) (16.0916, -1.5483) (16.1422, -1.5258) (16.1928, -1.5028) (16.2433, -1.4794) (16.2937, -1.4557) (16.3441, -1.4316) (16.3944, -1.4071) (16.4447, -1.3822) (16.4949, -1.3569) (16.545, -1.3313) (16.5951, -1.3053) (16.6451, -1.2789) (16.695, -1.2521) (16.7448, -1.225) (16.7946, -1.1975) (16.8443, -1.1697) (16.8939, -1.1415) (16.9435, -1.1129) (16.9929, -1.084) (17.0423, -1.0548) (17.0916, -1.0251) (17.1408, -0.9952) (17.1899, -0.9649) (17.239, -0.9343) (17.2879, -0.9033) (17.3368, -0.8719) (17.3856, -0.8403) (17.4245, -0.8147) (17.4537, -0.7953) (17.4731, -0.7824) (17.4828, -0.7759) knots 0 0 0 0 0 0 0.01428571 0.02857143 0.04285714 0.05714286 0.07142857 0.08571429 0.1 0.11428571 0.12857143 0.14285714 0.15714286 0.17142857 0.18571429 0.2 0.21428571 0.22857143 0.24285714 0.25714286 0.27142857 0.28571429 0.3 0.31428571 0.32857143 0.34285714 0.35714286 0.37142857 0.38571429 0.4 0.41428571 0.42857143 0.44285714 0.45714286 0.47142857 0.48571429 0.5 0.51428571 0.52857143 0.54285714 0.55714286 0.57142857 0.58571429 0.6 0.61428571 0.62857143 0.64285714 0.65714286 0.67142857 0.68571429 0.7 0.71428571 0.72857143 0.74285714 0.75714286 0.77142857 0.78571429 0.8 0.81428571 0.82857143 0.84285714 0.85714286 0.87142857 0.88571429 0.9 0.91428571 0.92857143 0.94285714 0.95714286 0.97142857 0.98571429 1 1 1 1 1 1
  spline S1 degree 5 poles (13.9458, 2.0479) (13.9559, 2.0494) (13.9759, 2.052) (14.0061, 2.0549) (14.0465, 2.057) (14.0972, 2.0572) (14.1481, 2.0556) (14.199, 2.0528) (14.2501, 2.0495) (14.3011, 2.0457) (14.3522, 2.0415) (14.4034, 2.0367) (14.4546, 2.0311) (14.5058, 2.0247) (14.5571, 2.0173) (14.6084, 2.0091) (14.6597, 2.0003) (14.7111, 1.9908) (14.7624, 1.9808) (14.8137, 1.9703) (14.8651, 1.9594) (14.9164, 1.9479) (14.9678, 1.9358) (15.0191, 1.9232) (15.0705, 1.91) (15.1218, 1.8963) (15.1731, 1.882) (15.2244, 1.8673) (15.2757, 1.8521) (15.3269, 1.8365) (15.3781, 1.8204) (15.4293, 1.8038) (15.4805, 1.7868) (15.5316, 1.7693) (15.5827, 1.7513) (15.6338, 1.7329) (15.6848, 1.7141) (15.7358, 1.6948) (15.7868, 1.6751) (15.8377, 1.655) (15.8886, 1.6345) (15.9394, 1.6136) (15.9902, 1.5922) (16.0409, 1.5705) (16.0916, 1.5483) (16.1422, 1.5258) (16.1928, 1.5028) (16.2433, 1.4794) (16.2937, 1.4557) (16.3441, 1.4316) (16.3944, 1.4071) (16.4447, 1.3822) (16.4949, 1.3569) (16.545, 1.3313) (16.5951, 1.3053) (16.6451, 1.2789) (16.695, 1.2521) (16.7448, 1.225) (16.7946, 1.1975) (16.8443, 1.1697) (16.8939, 1.1415) (16.9435, 1.1129) (16.9929, 1.084) (17.0423, 1.0548) (17.0916, 1.0251) (17.1408, 0.9952) (17.1899, 0.9649) (17.239, 0.9343) (17.2879, 0.9033) (17.3368, 0.8719) (17.3856, 0.8403) (17.4245, 0.8147) (17.4537, 0.7953) (17.4731, 0.7824) (17.4828, 0.7759) knots 0 0 0 0 0 0 0.01428571 0.02857143 0.04285714 0.05714286 0.07142857 0.08571429 0.1 0.11428571 0.12857143 0.14285714 0.15714286 0.17142857 0.18571429 0.2 0.21428571 0.22857143 0.24285714 0.25714286 0.27142857 0.28571429 0.3 0.31428571 0.32857143 0.34285714 0.35714286 0.37142857 0.38571429 0.4 0.41428571 0.42857143 0.44285714 0.45714286 0.47142857 0.48571429 0.5 0.51428571 0.52857143 0.54285714 0.55714286 0.57142857 0.58571429 0.6 0.61428571 0.62857143 0.64285714 0.65714286 0.67142857 0.68571429 0.7 0.71428571 0.72857143 0.74285714 0.75714286 0.77142857 0.78571429 0.8 0.81428571 0.82857143 0.84285714 0.85714286 0.87142857 0.88571429 0.9 0.91428571 0.92857143 0.94285714 0.95714286 0.97142857 0.98571429 1 1 1 1 1 1
  arc A0 (17.4828, -0.7759) -> (17.4828, 0.7759) centre (0, 0) ccw
  line L0 (11.8125, -1.7361) -> (13.9458, -2.0479)
  line L1 (11.8125, 1.7361) -> (13.9458, 2.0479)
  line L2 (11.8125, -1.7361) -> (11.8125, 1.7361)
  point P0 (14.1908, -2.0531)
  point P1 (14.4394, -2.0327)
  point P2 (14.6902, -1.9946)
  point P3 (14.9425, -1.9417)
  point P4 (15.196, -1.8754)
  point P5 (15.4504, -1.7967)
  point P6 (15.7053, -1.7063)
  point P7 (15.9604, -1.6047)
  point P8 (16.2156, -1.4922)
  point P9 (16.4704, -1.3692)
  point P10 (16.7248, -1.2358)
  point P11 (16.9785, -1.0924)
  point P12 (17.2312, -0.939)
  point P13 (14.1908, 2.0531)
  point P14 (14.4394, 2.0327)
  point P15 (14.6902, 1.9946)
  point P16 (14.9425, 1.9417)
  point P17 (15.196, 1.8754)
  point P18 (15.4504, 1.7967)
  point P19 (15.7053, 1.7063)
  point P20 (15.9604, 1.6047)
  point P21 (16.2156, 1.4922)
  point P22 (16.4704, 1.3692)
  point P23 (16.7248, 1.2358)
  point P24 (16.9785, 1.0924)
  point P25 (17.2312, 0.939)
extrude "돌출2''" add sketch "스케치2 (5)" along normal blind 5 bodies 5 in component "Spur Gear (12 teeth) (1) (1)"
fillet "필렛1'" radius 1 2 edges at (11.8222, -1.7375, 2.5) (11.8222, 1.7375, 2.5) on bodies 5 in component "Spur Gear (12 teeth) (1) (1)"
pattern_circular "C-패턴1'" count 6 over 150 about axis through (0, 0, 0) along (0, 0, 1) of "돌출2''", "필렛1'" in component "Spur Gear (12 teeth) (1) (1)"
sketch "스케치3 (5)" plane through (0, 0, 0) normal (0, 0, 1) x (1, 0, 0) in component "Spur Gear (12 teeth) (1) (1)"
  circle A0 centre (0, 0) radius 15 construction
sketch "스케치4 (2)" plane through (0, 0, 0) normal (0, 0, 1) x (1, 0, 0) in component "TRGRIP01_GearLink_Right"
  line L0 (-10, -4) -> (-50, -4)
  line L1 (-50, -4) -> (-50, 4)
  line L2 (-50, 4) -> (-10, 4)
  line L3 (-10, 4) -> (-10, -4)
  dimension "d35" = 50
  dimension "d36" = 40
  dimension "d37" = 8
  dimension "d38_1" = 4
  constraint horizontal L0
  constraint vertical L1
  constraint horizontal L2
  constraint vertical L3
  measures "d35" distance of L1 origin
  measures "d36" distance of L1.end L2.end
  measures "d37" distance of L0.end L1.end
  measures "d38_1" vertical distance of L1.end origin
extrude "돌출5" add sketch "스케치4 (2)" along normal blind 15 sketch seen with x (-0.965926, 0.258819, 0) y (-0.258819, -0.965926, 0) z (0, 0, 1) at (0, 0, 0) bodies 5 in component "Spur Gear (12 teeth) (1) (1)"
extrude "돌출7'" cut 1 faces at (9.3142, -3.8761, 8.3333) along direction (0.965926, -0.258819, 0) blind 10 on bodies 5 bodies 5 in component "Spur Gear (12 teeth) (1) (1)"
sketch "스케치10 (2)" plane through (0, -4, 0) normal (0, -1, 0) x (1, 0, 0) in component "TRGRIP01_GearLink_Right"
  line L0 (-50, 15) -> (-20, 15)
  line L1 (-20, 15) -> (-20, 0)
  line L2 (-20, 0) -> (-50, 0)
  line L3 (-50, 0) -> (-50, 15)
  line L4 (-17.0367, 0) -> (-50, 0)
  point P0 (-50, 15)
  constraint horizontal L0
  constraint vertical L1
  constraint horizontal L2
  constraint vertical L3
  constraint coincident L1.end L4
  constraint coincident P0 L0.start
extrude "돌출13''" add sketch "스케치10 (2)" along normal blind 6 sketch seen with x (-0.965926, 0.258819, 0) y (-0.258819, -0.965926, 0) z (0, 0, 1) at (0, 0, 0) bodies 5 in component "Spur Gear (12 teeth) (1) (1)"
chamfer "챔퍼4'" distance 10 angle 45 2 edges at (48.2963, -12.941, 15) (50.108, -6.1795, 15) on bodies 5 in component "Spur Gear (12 teeth) (1) (1)"
sketch "스케치6" plane through (0, 0, 5) normal (0, 0, 1) x (-1, 0, 0) in component "TRGRIP01_GearLink_Right"
  line L0 (16.5902, -2.3924) -> (0.2933, -3.6884)
  line L1 (16.5902, 2.3924) -> (0.2933, 3.6884)
  arc A0 (16.5902, -2.3924) -> (16.5902, 2.3924) centre (16.4, 0) ccw
  arc A1 (0.2933, 3.6884) -> (0.2933, -3.6884) centre (0, 0) ccw
  line L2 (5.3, -3.2902) -> (5.3, 3.2902)
  dimension "d48_1" = 7.4
  dimension "d49" = 4.8
  dimension "d50_1" = 16.4
  dimension "d51" = 5.3
  constraint coincident A1.centre origin
  constraint coincident L1.end A1
  constraint tangent L0 A0
  constraint tangent L0 A1
  constraint equal L0 L1
  constraint coincident L1 A1.start
  constraint horizontal A1.centre A0.centre
  constraint tangent L1 A0
  constraint tangent L1 A1
  constraint coincident L0 L2.start
  constraint coincident L1 L2.end
  constraint vertical L2
  measures "d48_1" diameter of A1
  measures "d49" diameter of A0
  measures "d50_1" distance of A1.centre A0.centre
  measures "d51" distance of A1.centre L2
extrude "돌출8'" cut sketch "스케치6" against normal blind 1.6 contours L0 L1 A0 L2 sketch seen with x (-0.965926, 0.258819, 0) y (-0.258819, -0.965926, 0) z (0, 0, 1) at (0, 0, 0) bodies 5 in component "Spur Gear (12 teeth) (1) (1)"
extrude "돌출9" cut sketch "스케치6" against normal blind 3.2 contours L0 L1 A1 L2 sketch seen with x (-0.965926, 0.258819, 0) y (-0.258819, -0.965926, 0) z (0, 0, 1) at (0, 0, 0) bodies 5 in component "Spur Gear (12 teeth) (1) (1)"
chamfer "챔퍼3" distance 1.6 angle 45 1 edges at (5.1194, -1.3717, 3.4) on bodies 5 in component "Spur Gear (12 teeth) (1) (1)"
sketch "스케치11 (2)" plane through (0, 0, 5) normal (0, 0, 1) x (-1, 0, 0) in component "TRGRIP01_GearLink_Right"
  circle A0 centre (0, 20) radius 26.5101
  arc A1 (-11.9403, 0.4615) -> (11.2598, -4) centre (0, 0) ccw
  point P0 (11.2598, -4)
  dimension "d70" = 20
  constraint vertical A1.centre A0.centre
  constraint coincident A0 P0
  measures "d70" distance of A1.centre A0.centre
extrude "돌출14'" cut sketch "스케치11 (2)" against normal blind 5 contours A0 A1 sketch seen with x (-0.965926, 0.258819, 0) y (-0.258819, -0.965926, 0) z (0, 0, 1) at (0, 0, 0) bodies 5 in component "Spur Gear (12 teeth) (1) (1)"
sketch "스케치12" plane through (0, 0, 0) normal (0, 0, -1) x (1, 0, 0) in component "TRGRIP01_GearLink_Right"
  circle A0 centre (-20, 50) radius 46
  circle A1 centre (-20, 50) radius 54
  line L0 (-50, -4) -> (-11.2598, -4)
  line L1 (-50, -4) -> (-20, -4)
  line L2 (-50, -4) -> (-50, 5.1001)
  line L3 (-20, 10) -> (-20, 4)
  line L4 (-20, 10) -> (-42.7156, 10)
  point P0 (-20, 4)
  point P1 (-50, -4)
  point P2 (-20, -4)
  point P3 (-20, 10)
  point P4 (-20, 10)
  dimension "d75" = 50
  dimension "d76" = 20
  constraint concentric A0 A1
  constraint coincident A0 P0
  constraint coincident P1 L0.start
  constraint coincident P2 L1.end
  constraint coincident A1 P2
  constraint coincident A1 L2.end
  constraint coincident P4 P3
  constraint coincident P0 L3.end
  constraint coincident A0 L4.end
  constraint perpendicular L3 L4
  measures "d75" vertical distance of A0.centre origin
  measures "d76" horizontal distance of A0.centre origin
extrude "돌출15'" cut sketch "스케치12" against normal blind 15 contours A0 L3 L4 | A1 L0 L1 L2 picked at (-21.9743, 6.1276) sketch seen with x (-0.965926, 0.258819, 0) y (-0.258819, -0.965926, 0) z (0, 0, 1) at (0, 0, 0) bodies 5 in component "Spur Gear (12 teeth) (1) (1)"
sketch "스케치1 (9)" plane through (0, 0, 0) normal (0, 0, 1) x (1, 0, 0) in component "TRGRIP01_Case_Top"
  line L0 (0, 0) -> (60, 0)
  line L1 (60, 0) -> (60, 30)
  line L2 (60, 30) -> (0, 30)
  line L3 (0, 30) -> (0, 0)
  dimension "d1_2" = 60
  dimension "d2_2" = 30
  constraint horizontal L0
  constraint vertical L1
  constraint horizontal L2
  constraint vertical L3
  constraint coincident L0.start L3.end
  measures "d1_2" distance of L0.start L0.end
  measures "d2_2" distance of L0.start L2.end
extrude "돌출1'''''" add sketch "스케치1 (9)" along normal blind 2 separate body makes body 6 in component "TRGRIP01_Case_Top"
sketch "스케치2 (6)" plane through (0, 0, 2) normal (0, 0, 1) x (-1, 0, 0) in component "TRGRIP01_Case_Top"
  circle A0 centre (-53.75, -8.1) radius 1.1
  circle A1 centre (-25.95, -8.1) radius 1.1
  circle A2 centre (-15, -8.1) radius 5
  line L0 (0, 0) -> (-60, 0)
  line L1 (-51.35, -2) -> (-51.35, -14.2)
  line L2 (-51.35, -14.2) -> (-28.35, -14.2)
  line L3 (-28.35, -14.2) -> (-28.35, -2)
  line L4 (-51.35, -2) -> (-28.35, -2)
  dimension "d5_1_1" = 2.2
  dimension "d6_1" = 27.8
  dimension "d8_1" = 8.1
  dimension "d9_3" = 10
  dimension "d11_3" = 15
  dimension "d28_1" = 25.95
  dimension "d91_1" = 23
  dimension "d93_1" = 2.4
  dimension "d94" = 2
  dimension "d95_1" = 12.2
  constraint equal A0 A1
  constraint horizontal A0.centre A1.centre
  constraint vertical L1
  constraint horizontal L2
  constraint vertical L3
  constraint horizontal A1.centre A2.centre
  constraint perpendicular L3 L4
  measures "d5_1_1" diameter of A0
  measures "d6_1" distance of A0.centre A1.centre
  measures "d8_1" vertical distance of L0.start A0.centre
  measures "d9_3" diameter of A2
  measures "d11_3" horizontal distance of L0.start A2.centre
  measures "d28_1" horizontal distance of L0.start A1.centre
  measures "d91_1" distance of L1 L3
  measures "d93_1" horizontal distance of A1.centre L3.end
  measures "d94" vertical distance of L0.start L1.start
  measures "d95_1" distance of L2.end L3.end
extrude "돌출2'''" cut sketch "스케치2 (6)" against normal blind 2 contours A0 | A1 | L1 L2 L3 L4 bodies 6 in component "TRGRIP01_Case_Top"